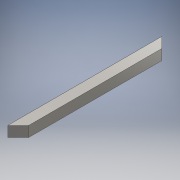
# Autodesk Inventor part: exterior support
Saved by Autodesk Inventor 2016 (Build 200138000, 138)
## iProperties
Created: 2019-03-25
Part Number: exterior support
Material: Stainless Steel
Document SubType Name: Modeling
Designer: benja
Density: 8 g/cm^3
Appearance: Semi-Polished
Author: benja
Autodesk Inventor part; units mm, degrees
ref_plane "YZ Plane" through (0, 0, 0) normal (1, 0, 0) x (0, 1, 0)
ref_plane "XZ Plane" through (0, 0, 0) normal (0, 1, 0) x (-1, 0, 0)
ref_plane "XY Plane" through (0, 0, 0) normal (0, 0, 1) x (1, 0, 0)
sketch "Sketch1" plane through (0, 0, 0) normal (0, 0, 1) x (1, 0, 0)
  line L0 (140, 140) -> (140, 1920)
  line L1 (0, 2060) -> (0, 0)
  line L2 (0, 2060) -> (140, 1920)
  line L3 (0, 2060) -> (197.9899, 2060) construction
  line L4 (0, 0) -> (140, 140)
  line L5 (0, 0) -> (197.9899, 0) construction
  dimension "d2" = 45
  dimension "d3" = 45
  constraints: 12 end point, 2 equal length, 2 horizontal, 1 parallel
  measures "d2" angle of L2 L3
  measures "d3" angle of L5 L4
extrude "Extrusion1" add sketch "Sketch1" along normal blind 140
body "Solid1"
